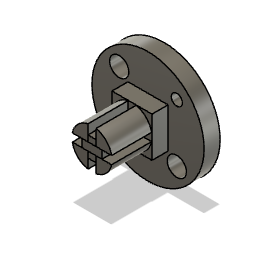
slotted_circle_peg_V2 v3 (Autodesk Fusion 360 design; units mm, degrees)
Autodesk Fusion 360 part; units mm, degrees
note: some values were not read from the file. Chosen so that the rebuilt part matches the saved one: which bodies a step acts on.
sketch "Sketch1" plane through (0, 0, 0) normal (0, 0, 1) x (1, 0, 0)
  circle A0 centre (0, 0) radius 35
  circle A1 centre (18, 18) radius 3.5
  circle A2 centre (-18, 18) radius 6
  circle A3 centre (-18, -18) radius 3.5
  circle A4 centre (18, -18) radius 6
  dimension "d1" = 70
  dimension "d2" = 7
  dimension "d3" = 18
  dimension "d4" = 18
  dimension "d5" = 12
  dimension "d6" = 18
  dimension "d7" = 18
  dimension "d8" = 7
  dimension "d9" = 18
  dimension "d10" = 18
  dimension "d11" = 12
  dimension "d12" = 18
  dimension "d13" = 18
  constraint coincident A0.centre origin
  measures "d1" diameter of A0
  measures "d2" diameter of A1
  measures "d3" horizontal distance of A0.centre A1.centre
  measures "d4" vertical distance of A0.centre A1.centre
  measures "d5" diameter of A2
  measures "d6" horizontal distance of A0.centre A2.centre
  measures "d7" vertical distance of A0.centre A2.centre
  measures "d8" diameter of A3
  measures "d9" vertical distance of A0.centre A3.centre
  measures "d10" horizontal distance of A0.centre A3.centre
  measures "d11" diameter of A4
  measures "d12" horizontal distance of A0.centre A4.centre
  measures "d13" vertical distance of A0.centre A4.centre
extrude "Extrude1" add sketch "Sketch1" against normal blind 10 makes body 1
sketch "Sketch2" plane through (0, 0, 0) normal (0, 0, 1) x (1, 0, 0)
  line L0 (12.5, 12.5) -> (-12.5, 12.5)
  line L1 (-12.5, 12.5) -> (-12.5, -12.5)
  line L2 (-12.5, -12.5) -> (12.5, -12.5)
  line L3 (12.5, -12.5) -> (12.5, 12.5)
  line L4 (12.5, 12.5) -> (-12.5, -12.5) construction
  line L5 (-12.5, 12.5) -> (12.5, -12.5) construction
  dimension "d16" = 25
  dimension "d17" = 25
  constraint horizontal L0
  constraint perpendicular L0 L1
  constraint parallel L0 L2
  constraint parallel L1 L3
  constraint coincident L4 origin
  constraint coincident L5 origin
  measures "d16" distance of L1.end L2.end
  measures "d17" distance of L0.start L2.end
extrude "Extrude2" add sketch "Sketch2" along normal blind 10 bodies 1
sketch "Sketch3" plane through (0, 0, 10) normal (0, 0, 1) x (1, 0, 0)
  line L0 (12.5, -12.5) -> (12.5, 12.5)
  line L1 (12.5, 12.5) -> (-12.5, 12.5)
  line L2 (-12.5, 12.5) -> (-12.5, -12.5)
  line L3 (-12.5, -12.5) -> (12.5, -12.5)
  circle A0 centre (0, 0) radius 12.5
  line L4 (6.25, 2.5) -> (18.75, 2.5)
  line L5 (18.75, 2.5) -> (18.75, -2.5)
  line L6 (18.75, -2.5) -> (6.25, -2.5)
  line L7 (6.25, -2.5) -> (6.25, 2.5)
  line L8 (6.25, 2.5) -> (18.75, -2.5) construction
  line L9 (18.75, 2.5) -> (6.25, -2.5) construction
  line L10 (2.5, 6.25) -> (-2.5, 6.25)
  line L11 (-2.5, 6.25) -> (-2.5, 18.75)
  line L12 (2.5, 18.75) -> (2.5, 6.25)
  line L13 (-2.5, 18.75) -> (2.5, 18.75)
  line L14 (-6.25, 2.5) -> (-6.25, -2.5)
  line L15 (-6.25, -2.5) -> (-18.75, -2.5)
  line L16 (-18.75, 2.5) -> (-6.25, 2.5)
  line L17 (-18.75, -2.5) -> (-18.75, 2.5)
  line L18 (-2.5, -6.25) -> (2.5, -6.25)
  line L19 (2.5, -6.25) -> (2.5, -18.75)
  line L20 (-2.5, -18.75) -> (-2.5, -6.25)
  line L21 (2.5, -18.75) -> (-2.5, -18.75)
  point P0 (12.5, 0)
  dimension "d20" = 5
  dimension "d21" = 6.25
  dimension "d23" = 360
  constraint coincident A0.centre origin
  constraint tangent L0 A0
  constraint horizontal L4
  constraint perpendicular L4 L5
  constraint parallel L4 L6
  constraint parallel L5 L7
  constraint coincident L8 P0
  constraint coincident L9 P0
  constraint midpoint L0 P0
  measures "d20" distance of L4.end L5.end
  measures "d21" distance of A0.centre L7
extrude "Extrude3" add sketch "Sketch3" along normal blind 25 contours A0 L4 L6 L7 L10 L11 L12 L14 L15 L16 L18 L19 L20 bodies 1
split "Split1" by plane through (0, 0, 0) normal (0, 0, 1) bodies 1 makes body 2 at (2.0833, 0.8333, 35)
split "Split2" by plane through (0, 0, 10) normal (0, 0, 1) bodies 2 makes body 3 at (2.0833, 0.8333, 35)
split "Split3" by plane through (6.25, 2.5, 10) normal (0, -1, 0) and through (12.2474, -2.5, 10) normal (0, 1, 0) bodies 3 makes body 4 at (9.2584, -8.3984, 26.6667) makes body 5 at (6.25, -0.8333, 18.3333)
split "Split4" by plane through (-2.5, 6.25, 10) normal (1, 0, 0) and through (2.5, 12.2474, 10) normal (-1, 0, 0) bodies 3 4 makes body 8 at (9.2584, -8.3984, 26.6667) makes body 9 at (-0.8333, -2.5, 18.3333) makes body 6 at (6.962, 10.3818, 26.6667) makes body 7 at (0.8333, 6.25, 18.3333)
equation "d21 = ( ( 13.5 / 2 ) - 0.5 ) * 1 mm"
